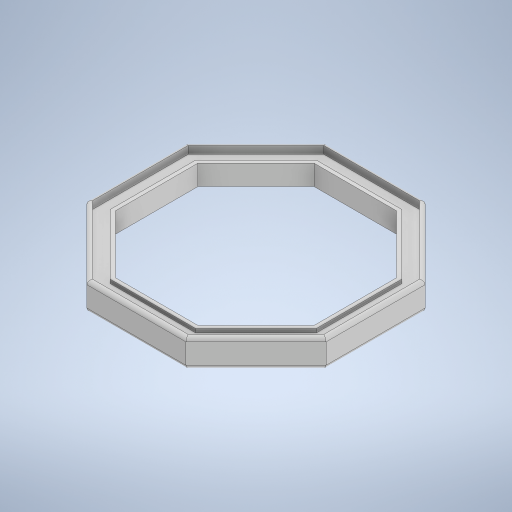
# Autodesk Inventor part: OV-PAM_ring_2
Saved by Autodesk Inventor 2024 (Build 280153000, 153)
## iProperties
Created: 2023-06-19
Part Number: OV-PAM_ring_2
Material: 일반
Document SubType Name: Modeling
Designer: jsw
Density: 1 g/cm^3
Appearance: 기본값
Author: jsw
Autodesk Inventor part; units mm, degrees
ref_plane "YZ Plane" through (0, 0, 0) normal (1, 0, 0) x (0, 1, 0)
ref_plane "XZ Plane" through (0, 0, 0) normal (0, 1, 0) x (-1, 0, 0)
sketch "스케치1" plane through (0, 0, 0) normal (0, 1, 0) x (-1, 0, 0)
  line L0 (-16.2959, 6.75) -> (-6.75, 16.2959)
  line L1 (-6.75, 16.2959) -> (6.75, 16.2959)
  line L2 (6.75, 16.2959) -> (16.2959, 6.75)
  line L3 (16.2959, 6.75) -> (16.2959, -6.75)
  line L4 (16.2959, -6.75) -> (6.75, -16.2959)
  line L5 (6.75, -16.2959) -> (-6.75, -16.2959)
  line L6 (-6.75, -16.2959) -> (-16.2959, -6.75)
  line L7 (-16.2959, -6.75) -> (-16.2959, 6.75)
  line L8 (18.8959, 7.827) -> (18.8959, -7.827)
  line L9 (18.8959, -7.827) -> (7.827, -18.8959)
  line L10 (7.827, -18.8959) -> (-7.827, -18.8959)
  line L11 (-7.827, -18.8959) -> (-18.8959, -7.827)
  line L12 (-18.8959, -7.827) -> (-18.8959, 7.827)
  line L13 (-18.8959, 7.827) -> (-7.827, 18.8959)
  line L14 (-7.827, 18.8959) -> (7.827, 18.8959)
  line L15 (7.827, 18.8959) -> (18.8959, 7.827)
  point P0 (0, 0)
  point P1 (0, 0)
  point P2 (0, 0)
  dimension "d0" = 13.5
  dimension "d1" = 2.6
  constraints: 32 end point, 2 coincident, 2 horizontal, 34 other
  measures "d0" distance of L2.end L3.end
  measures "d1" distance between parallel lines of L8 L3
extrude "돌출1" add sketch "스케치1" along normal blind 4.4 contours L0 L1 L2 L3 L4 L5 L6 L7 | L8 L9 L10 L11 L12 L13 L14 L15
sketch "스케치14" plane through (0, 4.4, 0) normal (0, 1, 0) x (1, 0, 0)
  line L0 (6.75, -16.2959) -> (-6.75, -16.2959)
  line L1 (-6.75, -16.2959) -> (-16.2959, -6.75)
  line L2 (-16.2959, -6.75) -> (-16.2959, 6.75)
  line L3 (-16.2959, 6.75) -> (-6.75, 16.2959)
  line L4 (-6.75, 16.2959) -> (6.75, 16.2959)
  line L5 (6.75, 16.2959) -> (16.2959, 6.75)
  line L6 (16.2959, 6.75) -> (16.2959, -6.75)
  line L7 (16.2959, -6.75) -> (6.75, -16.2959)
  line L8 (-7.5784, 18.2959) -> (7.5784, 18.2959)
  line L9 (7.5784, 18.2959) -> (18.2959, 7.5784)
  line L10 (18.2959, 7.5784) -> (18.2959, -7.5784)
  line L11 (18.2959, -7.5784) -> (7.5784, -18.2959)
  line L12 (7.5784, -18.2959) -> (-7.5784, -18.2959)
  line L13 (-7.5784, -18.2959) -> (-18.2959, -7.5784)
  line L14 (-18.2959, -7.5784) -> (-18.2959, 7.5784)
  line L15 (-18.2959, 7.5784) -> (-7.5784, 18.2959)
  line L16 (18.8959, -7.827) -> (18.8959, 7.827) projected
  point P0 (0, 0)
  point P1 (0, 0)
  point P2 (0, 0)
  dimension "d138" = 2
  dimension "d139" = 0.6
  constraints: 32 end point, 2 coincident, 2 horizontal, 34 other
  measures "d138" distance between parallel lines of L10 L6
  measures "d139" distance between parallel lines of L10 L16
extrude "돌출16" cut sketch "스케치14" against normal blind 1.2
sketch "스케치15" plane through (0, 4.4, 0) normal (0, 1, 0) x (1, 0, 0)
  line L0 (-16.2959, -6.75) -> (-6.75, -16.2959) projected
  line L1 (-6.75, -16.2959) -> (6.75, -16.2959) projected
  line L2 (6.75, -16.2959) -> (16.2959, -6.75) projected
  line L3 (16.2959, -6.75) -> (16.2959, 6.75) projected
  line L4 (16.2959, 6.75) -> (6.75, 16.2959) projected
  line L5 (6.75, 16.2959) -> (-6.75, 16.2959) projected
  line L6 (-6.75, 16.2959) -> (-16.2959, 6.75) projected
  line L7 (-16.2959, 6.75) -> (-16.2959, -6.75) projected
  point P0 (0, 0)
extrude "돌출17" cut sketch "스케치15" against normal blind 0.6
sketch "스케치16" plane through (0, 3.8, 0) normal (0, 1, 0) x (1, 0, 0)
  line L0 (-6.5015, 15.6959) -> (6.5015, 15.6959)
  line L1 (6.5015, 15.6959) -> (15.6959, 6.5015)
  line L2 (15.6959, 6.5015) -> (15.6959, -6.5015)
  line L3 (15.6959, -6.5015) -> (6.5015, -15.6959)
  line L4 (6.5015, -15.6959) -> (-6.5015, -15.6959)
  line L5 (-6.5015, -15.6959) -> (-15.6959, -6.5015)
  line L6 (-15.6959, -6.5015) -> (-15.6959, 6.5015)
  line L7 (-15.6959, 6.5015) -> (-6.5015, 15.6959)
  line L8 (16.2959, 6.75) -> (16.2959, -6.75) projected
  point P0 (0, 0)
  point P1 (0, 0)
  dimension "d144" = 0.6
  constraints: 16 end point, 1 coincident, 1 horizontal, 17 other
  measures "d144" distance between parallel lines of L2 L8
extrude "돌출18" cut sketch "스케치16" against normal up to surface (3.8 mm away)
fillet "모깎기2" radius 0.6 16 edges at (0, 4.4, -18.8959) (-13.3614, 4.4, -13.3614) (13.3614, 4.4, -13.3614) (18.8959, 4.4, 0) (13.3614, 4.4, 13.3614) (0, 4.4, 18.8959) (-13.3614, 4.4, 13.3614) (-18.8959, 4.4, 0) (-18.8959, 0, 0) (-13.3614, 0, 13.3614) (0, 0, 18.8959) (13.3614, 0, 13.3614) (-13.3614, 0, -13.3614) (0, 0, -18.8959) (18.8959, 0, 0) (13.3614, 0, -13.3614)
ref_plane "작업 평면3" through (0, 2.2, 0) normal (0, -1, 0) x (1, 0, 0)
mirror "미러6" about plane through (0, 2.2, 0) normal (0, -1, 0) of "돌출17", "돌출16"
